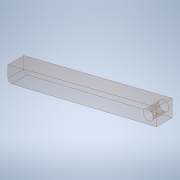
# Autodesk Inventor part: カウンター展開
Saved by Autodesk Inventor 2020.2 (Build 242310000, 310)
## iProperties
Created: 2020-04-03
Part Number: カウンター展開
Material: ポリカーボネート、スモーク
Document SubType Name: Modeling
Designer: aoyama
Density: 1.2 g/cm^3
Appearance: ポリカーボネート - スモーク
Mass: 1.30637 g
Surface Area: 11.931 cm^2
Volume: 1.08864 cm^3
Author: aoyama
Autodesk Inventor part; units mm, degrees
ref_plane "YZ Plane" through (0, 0, 0) normal (1, 0, 0) x (0, 1, 0)
ref_plane "XZ Plane" through (0, 0, 0) normal (0, 1, 0) x (-1, 0, 0)
ref_plane "XY Plane" through (0, 0, 0) normal (0, 0, 1) x (1, 0, 0)
sketch "スケッチ1" plane through (0, 0, 0) normal (0, 0, 1) x (1, 0, 0)
  line L0 (0, 0) -> (-100, 0) construction
  line L1 (0, 0) -> (-100, 0) construction
  line L2 (0, 5) -> (-100, 5)
  line L3 (-100, -5) -> (0, -5)
  arc A0 (0, -5) -> (0, 5) centre (0, 0) ccw
  circle A1 centre (0, 0) radius 1.5
  line L4 (-29.5, 1.5) -> (-29.5, 6.5)
  line L5 (-29.5, 1.5) -> (17.6, 12.9566)
  line L6 (17.6, 12.9566) -> (17.6, 18.3341)
  line L7 (17.6, 18.3341) -> (-29.5, 6.5)
  circle A2 centre (0, 15) radius 1.5
  line L8 (0, 15) -> (0, 0)
  circle A3 centre (0, 15) radius 2.5
  circle A4 centre (15, 15) radius 2.5
  circle A5 centre (15, 15) radius 1.5
  line L9 (-30, 6.8899) -> (-30, 0.8638)
  line L10 (-30, 0.8638) -> (18.1, 12.5637)
  line L11 (18.1, 12.5637) -> (18.1, 18.9752)
  line L12 (18.1, 18.9752) -> (-30, 6.8899)
  line L13 (-100, 5) -> (-100, -5)
  line L14 (0, 0) -> (-11, 0)
  line L15 (-11, 0) -> (-11, -3.5)
  line L16 (-11, 0) -> (-7.5, 0) construction
  line L17 (-11, -3.5) -> (0, -3.5)
  circle A6 centre (0, 0) radius 3.5
  line L18 (0, 5) -> (2.4995, 2.45)
  line L19 (-11, 0) -> (-11, -5)
  line L20 (15, 15) -> (15, 15)
  circle A7 centre (15, 15) radius 1.6
  circle A8 centre (15, 15) radius 2.6
  line L21 (-67.5, 5) -> (-67.5, -5)
  point P0 (-22.08, 5)
  point P1 (-39.5, 5)
  point P2 (0, 12.5)
  point P3 (0.6029, 12.5738)
  point P4 (0, 9.4363)
  point P5 (2.4999, 15.0163)
  point P6 (-2.3088, 14.0412)
  point P7 (-19.5417, 5)
  point P8 (-40, 5)
  point P9 (-11, -4.9654)
  dimension "d24" = 100
  dimension "d25" = 3
  dimension "d26" = 5
  dimension "d27" = 3
  dimension "d28" = 15
  dimension "d29" = 1
  dimension "d30" = 15
  dimension "d31" = 0.5
  dimension "d32" = 5
  dimension "d33" = 11
  dimension "d34" = 90
  dimension "d35" = 7
  dimension "d36" = 0
  dimension "d37" = 3.2
  dimension "d38" = 1
  dimension "d39" = 70
  dimension "d40" = 37.5
  dimension "d41" = 100
  dimension "d42" = 3.5
  constraints: 48 end point, 9 centre point, 7 tangent, 6 horizontal, 5 point on line, 5 vertical, 4 point on circle, 3 coincident, 1 parallel, 1 perpendicular, 7 other
  measures "d24" distance of L1.end L1.start
  measures "d25" diameter of A1
  measures "d26" distance of L4.start L4.end
  measures "d27" diameter of A2
  measures "d28" distance of L8.start L8.end
  measures "d29" radial gap between concentric circles of A2 A3
  measures "d30" distance of L8.start L20.start
  measures "d31" distance between parallel lines of L4 L9
  measures "d32" radius of A0
  measures "d33" distance of L14.end L8.end
  measures "d34" angle of L15 L16
  measures "d35" diameter of A6
  measures "d36" distance of L20.start L20.end
  measures "d37" diameter of A7
  measures "d38" radial gap between concentric circles of A7 A8
  measures "d39" distance from line of L2.end L9
  measures "d40" distance between parallel lines of L9 L21
  measures "d41" distance between parallel lines of L8 L13
  measures "d42" distance from line of L2 L4.start
extrude "押し出し1" add sketch "スケッチ1" along normal blind 5 contours L4 L7 A3 L8 L5 L2 | L2 L5 L4 | L8 A3 L7 A8 L5 | L7 A2 L8 A3 | A8 L6 L5 | A8 | L8 A2 L7 A3 | L7 L8 A2 | L7 L6 A8 | L8 L7 A2 | A4
fillet "フィレット1" radius 1 1 edges at (-29.5, 1.5, 2.5)
